Autodesk Inventor part; units mm, degrees
(part 2 of 2)
extrude "Extrusion17" cut sketch "Sketch16" against normal through all contours L3 L12 A1 L13 A0 L9
ref_plane "Work Plane1" through (-93.3464, 7, 45.7) normal (0, 0, 1) x (1, 0, 0)
sketch "Sketch18" plane through (-93.3464, 7, 45.7) normal (0, 0, 1) x (1, 0, 0)
  line L0 (0, 0) -> (0, 43) projected
  line L1 (6.6464, 8) -> (6.6464, 43) projected
  line L2 (6.6464, 43) -> (6.6464, 8) projected
  line L3 (0, 43) -> (40.3464, 43) projected
  line L4 (6.6464, 43) -> (6.6464, 8) projected
  line L5 (40.3464, 43) -> (40.3464, 25.5) projected
  arc A0 (40.3464, 25.5) -> (45.8464, 20) centre (45.8464, 25.5) ccw projected
  line L6 (45.8464, 20) -> (120.8464, 20) projected
  arc A1 (120.8464, 20) -> (126.3464, 25.5) centre (120.8464, 25.5) ccw projected
  line L7 (126.3464, 25.5) -> (126.3464, 43) projected
  line L8 (166.6929, 43) -> (126.3464, 43) projected
  line L9 (166.6929, 0) -> (166.6929, 43) projected
  line L10 (0, 0) -> (166.6929, 0) projected
  line L11 (0, 0) -> (0, 43) projected
  line L12 (40.3464, 43) -> (0, 43) projected
  line L13 (40.3464, 43) -> (6.6464, 43) projected
  line L14 (40.3464, 43) -> (40.3464, 25.5) projected
  arc A2 (40.3464, 25.5) -> (45.8464, 20) centre (45.8464, 25.5) ccw projected
  line L15 (45.8464, 20) -> (120.8464, 20) projected
  arc A3 (120.8464, 20) -> (126.3464, 25.5) centre (120.8464, 25.5) ccw projected
  line L16 (126.3464, 25.5) -> (126.3464, 43) projected
  line L17 (160.0464, 43) -> (126.3464, 43) projected
  line L18 (160.0464, 8) -> (160.0464, 43) projected
  line L19 (6.6464, 8) -> (160.0464, 8) projected
  line L20 (6.6464, 43) -> (6.6464, 8) projected
  line L21 (40.3464, 43) -> (6.6464, 43) projected
  arc A4 (6.6464, 31.5862) -> (6.6464, 38.5862) centre (-0.5473, 35.0862) ccw
  point P0 (93.3464, -7)
  dimension "d259" = 7
  dimension "d260" = 8
  constraints: 2 point on circle, 2 point on line, 1 centre point
  measures "d259" distance of A4.end A4.start
  measures "d260" radius of A4
extrude "Extrusion18" add sketch "Sketch18" along normal mid plane 2 fills toward (7.4027, 35.0862) open curves A4
ref_plane "Work Plane2" through (-93.3464, 7, -0.05) normal (0, 0, 1) x (1, 0, 0)
ref_plane "Work Plane3" through (-10.002, 7, -25.95) normal (-1, 0, 0) x (0, 0, 1)
mirror "Mirror1" about plane through (-93.3464, 7, -0.05) normal (0, 0, 1) of "Extrusion18"
mirror "Mirror2" about plane through (-10.002, 7, -25.95) normal (-1, 0, 0) of "Extrusion18", "Mirror1"
body "Solid1"
